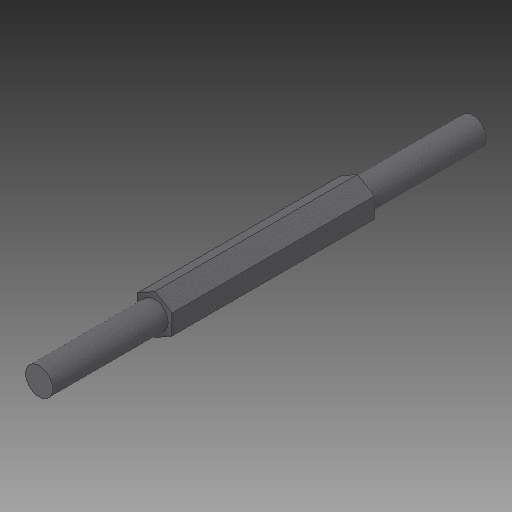
# Autodesk Inventor part: HexBar1Inch
Saved by Autodesk Inventor 2018 (Build 220112000, 112)
## iProperties
Created: 2018-01-21
Part Number: HexBar1Inch
Material: Generic
Document SubType Name: Modeling
Designer: Olivier
Density: 1 g/cm^3
Appearance: Default
Mass: 136.8 g
Surface Area: 249.316 cm^2
Volume: 136.8 cm^3
Author: Olivier
Autodesk Inventor part; units mm, degrees
ref_plane "YZ Plane" through (0, 0, 0) normal (1, 0, 0) x (0, 1, 0)
ref_plane "XZ Plane" through (0, 0, 0) normal (0, 1, 0) x (-1, 0, 0)
ref_plane "XY Plane" through (0, 0, 0) normal (0, 0, 1) x (1, 0, 0)
sketch "Sketch1" plane through (0, 0, 0) normal (0, 0, 1) x (1, 0, 0)
  line L0 (-12.6808, 7.3656) -> (0.0383, 14.6647)
  line L1 (0.0383, 14.6647) -> (12.7192, 7.2991)
  line L2 (12.7192, 7.2991) -> (12.6808, -7.3656)
  line L3 (12.6808, -7.3656) -> (-0.0383, -14.6647)
  line L4 (-0.0383, -14.6647) -> (-12.7192, -7.2991)
  line L5 (-12.7192, -7.2991) -> (-12.6808, 7.3656)
  point P0 (0, 0)
  dimension "d10" = 29.3294
  constraints: 12 end point, 13 other
  measures "d10" vertical distance of L3.end L0.end
extrude "Extrusion1" add sketch "Sketch1" along normal blind 149.255
sketch "Sketch2" plane through (0, 0, 0) normal (0, 0, -1) x (-1, 0, 0)
  circle A0 centre (0, 0) radius 10
  dimension "d13" = 20
  constraints: 1 centre point, 1 coincident
  measures "d13" diameter of A0
sketch "Sketch3" plane through (0, 0, 149.255) normal (0, 0, 1) x (1, 0, 0)
  circle A0 centre (0, 0) radius 10
  dimension "d14" = 20
  constraints: 1 centre point, 1 coincident
  measures "d14" diameter of A0
extrude "Extrusion2" add sketch "Sketch3" along normal blind 85
extrude "Extrusion3" add sketch "Sketch2" along normal blind 85
body "Solid1"
